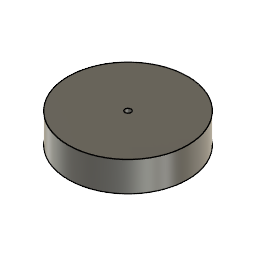
small_spur_gear_2 (Autodesk Fusion 360 design; units mm, degrees)
part number: 2025-11-09-11-34-01-978
part number: 2025-11-14-11-31-04-685
Autodesk Fusion 360 part; units mm, degrees
sketch "Sketch2" plane through (0, 0, 0) normal (0, 0, 1) x (1, 0, 0)
  circle A0 centre (0, 0) radius 20
  circle A1 centre (0, 0) radius 1
  dimension "d22" = 40
  constraint coincident A0.centre A1.centre
  measures "d22" diameter of A0
extrude "Extrude1" add sketch "Sketch2" along normal blind 10 makes body 1
copy_body "Body->Comp1" bodies 1 removing the originals makes body 2 in component "Component"
component "Component" placed x (1, 0, 0) y (0, 1, 0) z (0, 0, 1) at (0, 0, 0)
